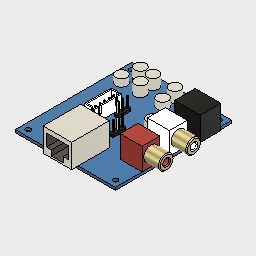
Rock64 ES9023 audio POT (Autodesk Fusion 360 design; units mm, degrees)
Autodesk Fusion 360 part; units mm, degrees
sketch "Sketch1" plane through (0, 0, 0) normal (0, 1, 0) x (1, 0, 0)
  line L0 (28.05, -32.6) -> (-28.05, -32.6)
  line L1 (-28.05, -32.6) -> (-28.05, 32.6)
  line L2 (-28.05, 32.6) -> (28.05, 32.6)
  line L3 (28.05, 32.6) -> (28.05, -32.6)
  line L4 (2.5, 0) -> (20, 0)
  line L5 (0, -20) -> (0, -2.5)
  circle A0 centre (-24.45, 29) radius 1.375
  circle A1 centre (24.55, 29) radius 1.375
  circle A2 centre (24.55, -29) radius 1.375
  circle A3 centre (-24.45, -29) radius 1.375
  dimension "d1" = 65.2
  dimension "d2" = 56.1
  dimension "d3" = 49
  dimension "d4" = 58
  dimension "d5" = 2.75
  dimension "d6" = 3.6
  dimension "d7" = 3.6
  measures "d1" distance of L0 L2
  measures "d2" distance of L1 L3
  measures "d3" distance of A0.centre A1.centre
  measures "d4" distance of A0.centre A3.centre
  measures "d5" diameter of A0
  measures "d6" distance of L0 A3.centre
  measures "d7" distance of L1 A3.centre
extrude "Extrude1" add sketch "Sketch1" along normal blind 1.5
sketch "Sketch2" plane through (0, 1.5, 0) normal (0, 1, 0) x (-1, 0, 0)
  circle A0 centre (24.45, 29) radius 1.375
  circle A1 centre (-24.55, 29) radius 1.375
  circle A2 centre (-24.55, -29) radius 1.375
  circle A3 centre (24.45, -29) radius 1.375
  line L0 (-28.05, -32.6) -> (28.05, -32.6)
  line L1 (28.05, -32.6) -> (28.05, 32.6)
  line L2 (28.05, 32.6) -> (-28.05, 32.6)
  line L3 (-28.05, 32.6) -> (-28.05, -32.6)
  line L4 (8.8, 15.2) -> (-7.2, 15.2)
  line L5 (-7.2, 15.2) -> (-7.2, 36.3)
  line L6 (-7.2, 36.3) -> (8.8, 36.3)
  line L7 (8.8, 36.3) -> (8.8, 15.2)
  dimension "d10" = 16
  dimension "d11" = 21.1
  dimension "d12" = 35.25
  dimension "d13" = 3.7
  measures "d10" distance of L5 L7
  measures "d11" distance of L4 L6
  measures "d12" distance of L1 L5
  measures "d13" distance of L2 L6
extrude "Extrude2" add sketch "Sketch2" along normal blind 13.25 contours L2 L5 L6 L7 | L2 L4 L5 L7
sketch "Sketch3" plane through (0, 0, 36.3) normal (0, 0, 1) x (1, 0, 0)
  line L0 (-8.8, 1.5) -> (7.2, 1.5)
  line L1 (7.2, 1.5) -> (7.2, 14.75)
  line L2 (7.2, 14.75) -> (-8.8, 14.75)
  line L3 (-8.8, 14.75) -> (-8.8, 1.5)
  line L4 (-6.8, 12.25) -> (5.2, 12.25)
  line L5 (5.2, 12.25) -> (5.2, 5.5)
  line L6 (-6.8, 5.5) -> (-6.8, 12.25)
  line L7 (2.5, 5.5) -> (2.5, 2.5)
  line L8 (2.5, 2.5) -> (-4.1, 2.5)
  line L9 (-4.1, 2.5) -> (-4.1, 5.5)
  line L10 (5.2, 5.5) -> (2.5, 5.5)
  line L11 (-4.1, 5.5) -> (-6.8, 5.5)
  dimension "d16" = 2.5
  dimension "d17" = 2
  dimension "d18" = 2
  dimension "d19" = 1
  dimension "d20" = 4
  dimension "d21" = 6.6
  measures "d16" distance of L2 L4
  measures "d17" distance of L3 L6
  measures "d18" distance of L1 L5
  measures "d19" distance of L0 L8
  measures "d20" distance of L0 L11
  measures "d21" distance of L7 L9
extrude "Extrude3" cut sketch "Sketch3" against normal blind 15 contours L4 L5 L6 L7 L8 L9 L10 L11
sketch "Sketch4" plane through (0, 1.5, 0) normal (0, 1, 0) x (-1, 0, 0)
  line L0 (-7.2, 15.2) -> (-7.2, 32.6)
  line L1 (-7.2, 32.6) -> (-28.05, 32.6)
  line L2 (-28.05, 32.6) -> (-28.05, -32.6)
  line L3 (-28.05, -32.6) -> (28.05, -32.6)
  line L4 (28.05, -32.6) -> (28.05, 32.6)
  line L5 (28.05, 32.6) -> (8.8, 32.6)
  line L6 (8.8, 32.6) -> (8.8, 15.2)
  line L7 (8.8, 15.2) -> (-7.2, 15.2)
  circle A0 centre (24.45, 29) radius 1.375
  circle A1 centre (-24.55, 29) radius 1.375
  circle A2 centre (-24.55, -29) radius 1.375
  circle A3 centre (24.45, -29) radius 1.375
  line L8 (-15.74, -7.7) -> (-28.04, -7.7)
  line L9 (-28.04, -7.7) -> (-28.04, 2.3)
  line L10 (-28.04, 2.3) -> (-15.74, 2.3)
  line L11 (-15.74, 2.3) -> (-15.74, -7.7)
  line L12 (-15.74, 7.6) -> (-28.04, 7.6)
  line L13 (-28.04, 7.6) -> (-28.04, 17.6)
  line L14 (-28.04, 17.6) -> (-15.74, 17.6)
  line L15 (-15.74, 17.6) -> (-15.74, 7.6)
  dimension "d24" = 12.3
  dimension "d25" = 10
  dimension "d26" = 5.3
  dimension "d27" = 15
  dimension "d30" = 0.01
  measures "d24" distance of L9 L11
  measures "d25" distance of L8 L10
  measures "d26" distance of L10 L12
  measures "d27" distance of L1 L14
  measures "d30" distance of L2 L9
extrude "Extrude4" add sketch "Sketch4" along normal blind 12.42 contours L8 L9 L10 L11 | L12 L13 L14 L15
sketch "Sketch5" plane through (28.04, 0, 0) normal (1, 0, 0) x (0, 0, -1)
  line L0 (-2.3, 1.5) -> (7.7, 1.5)
  line L1 (7.7, 1.5) -> (7.7, 13.92)
  line L2 (7.7, 13.92) -> (-2.3, 13.92)
  line L3 (-2.3, 13.92) -> (-2.3, 1.5)
  circle A0 centre (2.7, 8.02) radius 4.1
  circle A1 centre (-12.6, 8.02) radius 4.1
  circle A2 centre (-12.6, 8.02) radius 1.7
  circle A3 centre (2.7, 8.02) radius 1.7
  line L4 (-17.6, 1.5) -> (-17.6, 13.92)
  dimension "d31" = 8.2
  dimension "d32" = 3.4
  dimension "d33" = 5
  dimension "d34" = 5
  dimension "d35" = 5.9
  measures "d31" diameter of A1
  measures "d32" diameter of A2
  measures "d33" distance of A1.centre L4
  measures "d34" distance of L3 A0.centre
  measures "d35" distance of L2 A0.centre
extrude "Extrude5" add sketch "Sketch5" along normal blind 8.75 contours A0 | A1
fillet "Fillet1" radius 0.5 4 edges at (36.79, 6.5374, 16.4225) (36.79, 8.6347, 14.185) (36.79, 6.5374, 1.1225) (36.79, 8.6347, -1.115)
sketch "Sketch6" plane through (0, 1.5, 0) normal (0, 1, 0) x (-1, 0, 0)
  line L0 (-15.74, 17.6) -> (-15.74, 7.6)
  line L1 (-15.74, 7.6) -> (-28.04, 7.6)
  line L2 (-28.04, 7.6) -> (-28.04, 17.6)
  line L3 (-28.04, 17.6) -> (-15.74, 17.6)
  line L4 (-15.74, 2.3) -> (-15.74, -7.7)
  line L5 (-15.74, -7.7) -> (-28.04, -7.7)
  line L6 (-28.04, -7.7) -> (-28.04, 2.3)
  line L7 (-28.04, 2.3) -> (-15.74, 2.3)
  line L8 (-7.2, 15.2) -> (-7.2, 32.6)
  line L9 (-7.2, 32.6) -> (-28.05, 32.6)
  line L10 (-28.05, 32.6) -> (-28.05, -32.6)
  line L11 (-28.05, -32.6) -> (28.05, -32.6)
  line L12 (28.05, -32.6) -> (28.05, 32.6)
  line L13 (28.05, 32.6) -> (8.8, 32.6)
  line L14 (8.8, 32.6) -> (8.8, 15.2)
  line L15 (8.8, 15.2) -> (-7.2, 15.2)
  circle A0 centre (24.45, 29) radius 1.375
  circle A1 centre (-24.55, 29) radius 1.375
  circle A2 centre (-24.55, -29) radius 1.375
  circle A3 centre (24.45, -29) radius 1.375
  line L16 (-15.75, -24.5) -> (-30.05, -24.5)
  line L17 (-30.05, -24.5) -> (-30.05, -12.9)
  line L18 (-30.05, -12.9) -> (-15.75, -12.9)
  line L19 (-15.75, -12.9) -> (-15.75, -24.5)
  dimension "d39" = 11.6
  dimension "d40" = 14.3
  dimension "d41" = 2
  dimension "d42" = 8.1
  measures "d39" distance of L16 L18
  measures "d40" distance of L17 L19
  measures "d41" distance of L10 L17
  measures "d42" distance of L11 L16
extrude "Extrude6" add sketch "Sketch6" along normal blind 13.3 contours L10 L16 L18 L19 | L10 L16 L17 L18
sketch "Sketch7" plane through (0, 0, 0) normal (0, -1, 0) x (1, 0, 0)
  circle A0 centre (-24.45, 29) radius 1.375
  circle A1 centre (24.55, 29) radius 1.375
  circle A2 centre (24.55, -29) radius 1.375
  circle A3 centre (-24.45, -29) radius 1.375
  line L0 (-28.05, -32.6) -> (28.05, -32.6)
  line L1 (28.05, -32.6) -> (28.05, 32.6)
  line L2 (28.05, 32.6) -> (-28.05, 32.6)
  line L3 (-28.05, 32.6) -> (-28.05, -32.6)
  line L4 (-21.35, 20.3) -> (-16.45, 20.3)
  line L5 (-16.45, 20.3) -> (-16.45, -8.1)
  line L6 (-16.45, -8.1) -> (-21.35, -8.1)
  line L7 (-21.35, -8.1) -> (-21.35, 20.3)
  dimension "d45" = 4.9
  dimension "d46" = 28.4
  dimension "d47" = 6.7
  dimension "d48" = 12.3
  measures "d45" distance of L5 L7
  measures "d46" distance of L4 L6
  measures "d47" distance of L3 L7
  measures "d48" distance of L2 L4
extrude "Extrude7" add sketch "Sketch7" along normal blind 8.6 contours L4 L5 L6 L7
sketch "Sketch8" plane through (0, -8.6, 0) normal (0, -1, 0) x (1, 0, 0)
  line L0 (-21.35, -8.1) -> (-16.45, -8.1)
  line L1 (-16.45, -8.1) -> (-16.45, 20.3)
  line L2 (-16.45, 20.3) -> (-21.35, 20.3)
  line L3 (-21.35, 20.3) -> (-21.35, -8.1)
  line L4 (-20.49, 19.13) -> (-19.85, 19.13)
  line L5 (-19.85, 19.13) -> (-19.85, 18.49)
  line L6 (-19.85, 18.49) -> (-20.49, 18.49)
  line L7 (-20.49, 18.49) -> (-20.49, 19.13)
  dimension "d54" = 0.64
  dimension "d55" = 0.64
  dimension "d56" = 1.17
  dimension "d57" = 0.86
  measures "d54" distance of L4 L6
  measures "d55" distance of L5 L7
  measures "d56" distance of L2 L4
  measures "d57" distance of L3 L7
extrude "Extrude8" cut sketch "Sketch8" against normal blind 8 contours L4 L5 L6 L7
chamfer "Chamfer1" distance 0.55 angle 45 4 edges at (-19.85, -8.6, 18.81) (-20.17, -8.6, 19.13) (-20.49, -8.6, 18.81) (-20.17, -8.6, 18.49)
pattern_linear "R-Pattern1" count 2 spacing 2.54 along (1, 0, 0) count 11 spacing 2.54 along (0, 0, -1) of 9 faces at (-20.2767, -8.4167, 19.4967) (-20.8567, -8.4167, 18.9167) (-20.0633, -8.4167, 18.1233) (-19.4833, -8.4167, 18.9167) (-20.2767, -0.6, 18.9167) (-19.85, -5.5667, 18.9167) (-20.0633, -3.0833, 19.13) (-20.49, -5.5667, 18.7033) (-20.0633, -5.5667, 18.49)
sketch "Sketch9" plane through (0, 1.5, 0) normal (0, 1, 0) x (-1, 0, 0)
  line L0 (-15.75, -24.5) -> (-28.05, -24.5)
  line L1 (-28.05, -24.5) -> (-28.05, -32.6)
  line L2 (-28.05, -32.6) -> (28.05, -32.6)
  line L3 (28.05, -32.6) -> (28.05, 32.6)
  line L4 (28.05, 32.6) -> (8.8, 32.6)
  line L5 (8.8, 32.6) -> (8.8, 15.2)
  line L6 (8.8, 15.2) -> (-7.2, 15.2)
  line L7 (-7.2, 15.2) -> (-7.2, 32.6)
  line L8 (-7.2, 32.6) -> (-28.05, 32.6)
  line L9 (-28.05, 32.6) -> (-28.05, -12.9)
  line L10 (-28.05, -12.9) -> (-15.75, -12.9)
  line L11 (-15.75, -12.9) -> (-15.75, -24.5)
  line L12 (-15.74, 17.6) -> (-15.74, 7.6)
  line L13 (-15.74, 7.6) -> (-28.04, 7.6)
  line L14 (-28.04, 7.6) -> (-28.04, 17.6)
  line L15 (-28.04, 17.6) -> (-15.74, 17.6)
  line L16 (-15.74, 2.3) -> (-15.74, -7.7)
  line L17 (-15.74, -7.7) -> (-28.04, -7.7)
  line L18 (-28.04, -7.7) -> (-28.04, 2.3)
  line L19 (-28.04, 2.3) -> (-15.74, 2.3)
  circle A0 centre (24.45, 29) radius 1.375
  circle A1 centre (-24.55, 29) radius 1.375
  circle A2 centre (-24.55, -29) radius 1.375
  circle A3 centre (24.45, -29) radius 1.375
  line L20 (18.5, -7.46) -> (18.5, -5.72)
  line L21 (18.5, -5.72) -> (16.76, -5.72)
  line L22 (16.76, -5.72) -> (16.76, -7.46)
  line L23 (16.76, -7.46) -> (18.5, -7.46)
  line L24 (21.04, -7.46) -> (21.04, -5.72)
  line L25 (21.04, -5.72) -> (19.3, -5.72)
  line L26 (19.3, -5.72) -> (19.3, -7.46)
  line L27 (19.3, -7.46) -> (21.04, -7.46)
  line L28 (18.5, -4.92) -> (18.5, -3.18)
  line L29 (18.5, -3.18) -> (16.76, -3.18)
  line L30 (16.76, -3.18) -> (16.76, -4.92)
  line L31 (16.76, -4.92) -> (18.5, -4.92)
  line L32 (21.04, -4.92) -> (21.04, -3.18)
  line L33 (21.04, -3.18) -> (19.3, -3.18)
  line L34 (19.3, -3.18) -> (19.3, -4.92)
  line L35 (19.3, -4.92) -> (21.04, -4.92)
  line L36 (18.5, -2.38) -> (18.5, -0.64)
  line L37 (18.5, -0.64) -> (16.76, -0.64)
  line L38 (16.76, -0.64) -> (16.76, -2.38)
  line L39 (16.76, -2.38) -> (18.5, -2.38)
  line L40 (21.04, -2.38) -> (21.04, -0.64)
  line L41 (21.04, -0.64) -> (19.3, -0.64)
  line L42 (19.3, -0.64) -> (19.3, -2.38)
  line L43 (19.3, -2.38) -> (21.04, -2.38)
  line L44 (18.5, 0.16) -> (18.5, 1.9)
  line L45 (18.5, 1.9) -> (16.76, 1.9)
  line L46 (16.76, 1.9) -> (16.76, 0.16)
  line L47 (16.76, 0.16) -> (18.5, 0.16)
  line L48 (21.04, 0.16) -> (21.04, 1.9)
  line L49 (21.04, 1.9) -> (19.3, 1.9)
  line L50 (19.3, 1.9) -> (19.3, 0.16)
  line L51 (19.3, 0.16) -> (21.04, 0.16)
  line L52 (18.5, 2.7) -> (18.5, 4.44)
  line L53 (18.5, 4.44) -> (16.76, 4.44)
  line L54 (16.76, 4.44) -> (16.76, 2.7)
  line L55 (16.76, 2.7) -> (18.5, 2.7)
  line L56 (21.04, 2.7) -> (21.04, 4.44)
  line L57 (21.04, 4.44) -> (19.3, 4.44)
  line L58 (19.3, 4.44) -> (19.3, 2.7)
  line L59 (19.3, 2.7) -> (21.04, 2.7)
  line L60 (18.5, 5.24) -> (18.5, 6.98)
  line L61 (18.5, 6.98) -> (16.76, 6.98)
  line L62 (16.76, 6.98) -> (16.76, 5.24)
  line L63 (16.76, 5.24) -> (18.5, 5.24)
  line L64 (21.04, 5.24) -> (21.04, 6.98)
  line L65 (21.04, 6.98) -> (19.3, 6.98)
  line L66 (19.3, 6.98) -> (19.3, 5.24)
  line L67 (19.3, 5.24) -> (21.04, 5.24)
  line L68 (18.5, 7.78) -> (18.5, 9.52)
  line L69 (18.5, 9.52) -> (16.76, 9.52)
  line L70 (16.76, 9.52) -> (16.76, 7.78)
  line L71 (16.76, 7.78) -> (18.5, 7.78)
  line L72 (21.04, 7.78) -> (21.04, 9.52)
  line L73 (21.04, 9.52) -> (19.3, 9.52)
  line L74 (19.3, 9.52) -> (19.3, 7.78)
  line L75 (19.3, 7.78) -> (21.04, 7.78)
  line L76 (18.5, 10.32) -> (18.5, 12.06)
  line L77 (18.5, 12.06) -> (16.76, 12.06)
  line L78 (16.76, 12.06) -> (16.76, 10.32)
  line L79 (16.76, 10.32) -> (18.5, 10.32)
  line L80 (21.04, 10.32) -> (21.04, 12.06)
  line L81 (21.04, 12.06) -> (19.3, 12.06)
  line L82 (19.3, 12.06) -> (19.3, 10.32)
  line L83 (19.3, 10.32) -> (21.04, 10.32)
  line L84 (18.5, 12.86) -> (18.5, 14.6)
  line L85 (18.5, 14.6) -> (16.76, 14.6)
  line L86 (16.76, 14.6) -> (16.76, 12.86)
  line L87 (16.76, 12.86) -> (18.5, 12.86)
  line L88 (21.04, 12.86) -> (21.04, 14.6)
  line L89 (21.04, 14.6) -> (19.3, 14.6)
  line L90 (19.3, 14.6) -> (19.3, 12.86)
  line L91 (19.3, 12.86) -> (21.04, 12.86)
  line L92 (18.5, 15.4) -> (18.5, 17.14)
  line L93 (18.5, 17.14) -> (16.76, 17.14)
  line L94 (16.76, 17.14) -> (16.76, 15.4)
  line L95 (16.76, 15.4) -> (18.5, 15.4)
  line L96 (21.04, 15.4) -> (21.04, 17.14)
  line L97 (21.04, 17.14) -> (19.3, 17.14)
  line L98 (19.3, 17.14) -> (19.3, 15.4)
  line L99 (19.3, 15.4) -> (21.04, 15.4)
  line L100 (18.5, 17.94) -> (18.5, 19.68)
  line L101 (18.5, 19.68) -> (16.76, 19.68)
  line L102 (16.76, 19.68) -> (16.76, 17.94)
  line L103 (16.76, 17.94) -> (18.5, 17.94)
  line L104 (21.35, -8.1) -> (16.45, -8.1)
  line L105 (16.45, -8.1) -> (16.45, 20.3)
  line L106 (16.45, 20.3) -> (21.35, 20.3)
  line L107 (21.35, 20.3) -> (21.35, -8.1)
  line L108 (19.3, 19.68) -> (19.3, 17.94)
  line L109 (19.3, 17.94) -> (21.04, 17.94)
  line L110 (21.04, 17.94) -> (21.04, 19.68)
  line L111 (21.04, 19.68) -> (19.3, 19.68)
  circle A4 centre (20.17, -6.59) radius 0.635
  point P0 (20.17, -6.59)
  dimension "d77" = 1.27
  measures "d77" diameter of A4
extrude "Extrude10" add sketch "Sketch9" along normal blind 0.7 contours A4
fillet "Fillet4" radius 0.6 1 edges at (-19.578, 2.2, -6.8196)
pattern_linear "R-Pattern3" count 2 spacing 2.54 along (1, 0, 0) count 11 spacing 2.54 along (0, 0, 1) of 3 faces at (-20.1604, 2.2, -6.6) (-20.7491, 1.823, -6.4669) (-20.8042, 1.5667, -6.6217)
sketch "Sketch10" plane through (0, 1.5, 0) normal (0, 1, 0) x (-1, 0, 0)
  line L0 (8.5, 7.6) -> (14.25, 7.6)
  line L1 (14.25, 7.6) -> (14.25, -7.4)
  line L2 (14.25, -7.4) -> (8.5, -7.4)
  line L3 (8.5, -7.4) -> (8.5, 7.6)
  line L4 (28.05, -32.6) -> (28.05, 32.6)
  line L5 (28.05, 32.6) -> (8.8, 32.6)
  line L6 (13.5, -6.65) -> (9.25, -6.65)
  line L7 (9.25, -6.65) -> (9.25, 6.85)
  line L8 (9.25, 6.85) -> (13.5, 6.85)
  line L9 (13.5, 6.85) -> (13.5, -6.65)
  dimension "d83" = 0.75
  dimension "d104" = 15
  dimension "d105" = 5.75
  dimension "d106" = 13.8
  dimension "d107" = 25
  measures "d104" distance of L0 L2
  measures "d105" distance of L1 L3
  measures "d106" distance of L1 L4
  measures "d107" distance of L0 L5
extrude "Extrude11" add sketch "Sketch10" along normal blind 7.1
sketch "Sketch11" plane through (0, 1.5, 0) normal (0, 1, 0) x (-1, 0, 0)
  line L0 (9.25, 6.85) -> (9.25, -6.65)
  line L1 (9.25, -6.65) -> (13.5, -6.65)
  line L2 (13.5, -6.65) -> (13.5, 6.85)
  line L3 (13.5, 6.85) -> (9.25, 6.85)
  line L4 (11, -5.55) -> (10.35, -5.55)
  line L5 (10.35, -5.55) -> (10.35, -4.9)
  line L6 (10.35, -4.9) -> (11, -4.9)
  line L7 (11, -4.9) -> (11, -5.55)
  dimension "d86" = 1.1
  dimension "d87" = 0.65
  dimension "d88" = 0.65
  dimension "d89" = 1.1
  measures "d86" distance of L0 L5
  measures "d87" distance of L4.end L5.end
  measures "d88" distance of L4.start L4.end
  measures "d89" distance of L1 L4
extrude "Extrude12" add sketch "Sketch11" along normal blind 6.5 contours L4 L5 L6 L7
sketch "Sketch12" plane through (0, 8.6, 0) normal (0, 1, 0) x (-1, 0, 0)
  line L0 (9.25, 6.85) -> (13.5, 6.85)
  line L1 (13.5, 6.85) -> (13.5, -6.65)
  line L2 (13.5, -6.65) -> (9.25, -6.65)
  line L3 (9.25, -6.65) -> (9.25, 6.85)
  line L4 (8.5, -7.4) -> (14.25, -7.4)
  line L5 (14.25, -7.4) -> (14.25, 7.6)
  line L6 (14.25, 7.6) -> (8.5, 7.6)
  line L7 (8.5, 7.6) -> (8.5, -7.4)
  line L8 (9.25, -6.65) -> (10.35, -6.65)
  line L9 (10.35, -6.65) -> (10.35, -7.4)
  line L10 (10.35, -7.4) -> (9.25, -7.4)
  line L11 (9.25, -7.4) -> (9.25, -6.65)
  line L12 (9.25, -5.2) -> (8.5, -5.2)
  line L13 (8.5, -5.2) -> (8.5, -3.9)
  line L14 (8.5, -3.9) -> (9.25, -3.9)
  line L15 (9.25, -3.9) -> (9.25, -5.2)
  line L16 (8.5, 5.4) -> (9.25, 5.4)
  line L17 (9.25, 5.4) -> (9.25, 4.1)
  line L18 (9.25, 4.1) -> (8.5, 4.1)
  line L19 (8.5, 4.1) -> (8.5, 5.4)
  line L20 (9.25, 6.85) -> (10.35, 6.85)
  line L21 (10.35, 6.85) -> (10.35, 7.6)
  line L22 (10.35, 7.6) -> (9.25, 7.6)
  line L23 (9.25, 7.6) -> (9.25, 6.85)
  dimension "d92" = 1.1
  dimension "d93" = 1.1
  dimension "d94" = 2.2
  dimension "d95" = 1.3
  dimension "d96" = 2.2
  dimension "d97" = 1.3
  measures "d92" distance of L2.end L8.end
  measures "d93" distance of L21 L23
  measures "d94" distance of L6 L16
  measures "d95" distance of L16 L18
  measures "d96" distance of L4 L12
  measures "d97" distance of L12 L14
extrude "Extrude13" cut sketch "Sketch12" against normal blind 4 contours L0 L6 L20 L21 L22 L23 | L3 L7 L16 L17 L18 L19 | L3 L7 L12 L13 L14 L15 | L2 L4 L8 L9 L10 L11
pattern_linear "R-Pattern4" count 5 spacing 2.54 along (0, 0, 1) of "Extrude12"
sketch "Sketch14" plane through (0, 1.5, 0) normal (0, 1, 0) x (-1, 0, 0)
  circle A0 centre (24.45, -29) radius 1.375
  circle A1 centre (-24.55, -29) radius 1.375
  circle A2 centre (-24.55, 29) radius 1.375
  circle A3 centre (24.45, 29) radius 1.375
  line L0 (-15.74, 2.3) -> (-15.74, -7.7)
  line L1 (-15.74, -7.7) -> (-28.04, -7.7)
  line L2 (-28.04, -7.7) -> (-28.04, 2.3)
  line L3 (-28.04, 2.3) -> (-15.74, 2.3)
  line L4 (-15.74, 17.6) -> (-15.74, 7.6)
  line L5 (-15.74, 7.6) -> (-28.04, 7.6)
  line L6 (-28.04, 7.6) -> (-28.04, 17.6)
  line L7 (-28.04, 17.6) -> (-15.74, 17.6)
  line L8 (-15.75, -24.5) -> (-28.05, -24.5)
  line L9 (-28.05, -24.5) -> (-28.05, -32.6)
  line L10 (-28.05, -32.6) -> (28.05, -32.6)
  line L11 (28.05, -32.6) -> (28.05, 32.6)
  line L12 (28.05, 32.6) -> (8.8, 32.6)
  line L13 (8.8, 32.6) -> (8.8, 15.2)
  line L14 (8.8, 15.2) -> (-7.2, 15.2)
  line L15 (-7.2, 15.2) -> (-7.2, 32.6)
  line L16 (-7.2, 32.6) -> (-28.05, 32.6)
  line L17 (-28.05, 32.6) -> (-28.05, -12.9)
  line L18 (-28.05, -12.9) -> (-15.75, -12.9)
  line L19 (-15.75, -12.9) -> (-15.75, -24.5)
  circle A4 centre (20.17, -6.59) radius 0.635
  circle A5 centre (17.63, -6.59) radius 0.635
  circle A6 centre (20.17, -4.05) radius 0.635
  circle A7 centre (17.63, -4.05) radius 0.635
  circle A8 centre (20.17, -1.51) radius 0.635
  circle A9 centre (17.63, -1.51) radius 0.635
  circle A10 centre (20.17, 1.03) radius 0.635
  circle A11 centre (17.63, 1.03) radius 0.635
  circle A12 centre (20.17, 3.57) radius 0.635
  circle A13 centre (17.63, 3.57) radius 0.635
  circle A14 centre (20.17, 6.11) radius 0.635
  circle A15 centre (17.63, 6.11) radius 0.635
  circle A16 centre (20.17, 8.65) radius 0.635
  circle A17 centre (17.63, 8.65) radius 0.635
  circle A18 centre (20.17, 11.19) radius 0.635
  circle A19 centre (17.63, 11.19) radius 0.635
  circle A20 centre (20.17, 13.73) radius 0.635
  circle A21 centre (17.63, 13.73) radius 0.635
  circle A22 centre (20.17, 16.27) radius 0.635
  circle A23 centre (17.63, 16.27) radius 0.635
  circle A24 centre (20.17, 18.81) radius 0.635
  circle A25 centre (17.63, 18.81) radius 0.635
  line L20 (8.5, -7.4) -> (8.5, 7.6)
  line L21 (8.5, 7.6) -> (14.25, 7.6)
  line L22 (14.25, 7.6) -> (14.25, -7.4)
  line L23 (14.25, -7.4) -> (8.5, -7.4)
  line L24 (7.05, -9.1) -> (4.65, -9.1)
  line L25 (4.65, -9.1) -> (4.65, -1.32)
  line L26 (4.65, -1.32) -> (7.05, -1.32)
  line L27 (7.05, -1.32) -> (7.05, -9.1)
  line L28 (-0.95, 1.42) -> (-3.35, 1.42)
  line L29 (-3.35, 1.42) -> (-3.35, 9.2)
  line L30 (-3.35, 9.2) -> (-0.95, 9.2)
  line L31 (-0.95, 9.2) -> (-0.95, 1.42)
  dimension "d108" = 2.4
  dimension "d109" = 7.78
  dimension "d110" = 6
  dimension "d111" = 24.7
  dimension "d112" = 21
  dimension "d113" = 23.5
  measures "d108" distance of L25 L27
  measures "d109" distance of L24 L26
  measures "d110" distance of L14 L30
  measures "d111" distance of L17 L29
  measures "d112" distance of L11 L27
  measures "d113" distance of L10 L24
extrude "Extrude14" add sketch "Sketch14" along normal blind 1.3 contours L24 L25 L26 L27 | L28 L29 L30 L31
chamfer "Chamfer2" distance 0.65 angle 45 8 edges at (-7.05, 2.15, -9.1) (-4.65, 2.15, -9.1) (0.95, 2.15, 1.42) (3.35, 2.15, 1.42) (-7.05, 2.15, -1.32) (-4.65, 2.15, -1.32) (3.35, 2.15, 9.2) (0.95, 2.15, 9.2)
sketch "Sketch15" plane through (0, 2.8, 0) normal (0, 1, 0) x (-1, 0, 0)
  line L0 (5.3, -1.32) -> (4.65, -1.97)
  line L1 (4.65, -1.97) -> (4.65, -8.45)
  line L2 (4.65, -8.45) -> (5.3, -9.1)
  line L3 (5.3, -9.1) -> (6.4, -9.1)
  line L4 (6.4, -9.1) -> (7.05, -8.45)
  line L5 (7.05, -8.45) -> (7.05, -1.97)
  line L6 (7.05, -1.97) -> (6.4, -1.32)
  line L7 (6.4, -1.32) -> (5.3, -1.32)
  line L8 (6.17, -8.22) -> (5.52, -8.22)
  line L9 (5.52, -8.22) -> (5.52, -7.57)
  line L10 (5.52, -7.57) -> (6.17, -7.57)
  line L11 (6.17, -7.57) -> (6.17, -8.22)
  line L12 (-1.83, 2.3) -> (-2.48, 2.3)
  line L13 (-2.48, 2.3) -> (-2.48, 2.95)
  line L14 (-2.48, 2.95) -> (-1.83, 2.95)
  line L15 (-1.83, 2.95) -> (-1.83, 2.3)
  line L16 (-0.95, 2.07) -> (-0.95, 8.55)
  line L17 (-2.7, 1.42) -> (-1.6, 1.42)
  dimension "d117" = 0.65
  dimension "d118" = 0.88
  dimension "d119" = 0.88
  dimension "d120" = 0.88
  dimension "d121" = 0.88
  measures "d117" distance of L9 L11
  measures "d118" distance of L5 L11
  measures "d119" distance of L3 L8
  measures "d120" distance of L15 L16
  measures "d121" distance of L12 L17
extrude "Extrude15" add sketch "Sketch15" along normal blind 6 contours L8 L9 L10 L11 | L12 L13 L14 L15
pattern_linear "R-Pattern5" count 3 spacing 2.54 along (0, 0, 1) of "Extrude15"
sketch "Sketch16" plane through (0, 1.5, 0) normal (0, 1, 0) x (-1, 0, 0)
  line L0 (-0.95, 8.55) -> (-0.95, 2.07)
  line L1 (-0.95, 2.07) -> (-1.6, 1.42)
  line L2 (-1.6, 1.42) -> (-2.7, 1.42)
  line L3 (-2.7, 1.42) -> (-3.35, 2.07)
  line L4 (-3.35, 2.07) -> (-3.35, 8.55)
  line L5 (-3.35, 8.55) -> (-2.7, 9.2)
  line L6 (-2.7, 9.2) -> (-1.6, 9.2)
  line L7 (-1.6, 9.2) -> (-0.95, 8.55)
  line L8 (7.05, -1.97) -> (7.05, -8.45)
  line L9 (7.05, -8.45) -> (6.4, -9.1)
  line L10 (6.4, -9.1) -> (5.3, -9.1)
  line L11 (5.3, -9.1) -> (4.65, -8.45)
  line L12 (4.65, -8.45) -> (4.65, -1.97)
  line L13 (4.65, -1.97) -> (5.3, -1.32)
  line L14 (5.3, -1.32) -> (6.4, -1.32)
  line L15 (6.4, -1.32) -> (7.05, -1.97)
  circle A0 centre (24.45, -29) radius 1.375
  circle A1 centre (-24.55, -29) radius 1.375
  circle A2 centre (-24.55, 29) radius 1.375
  circle A3 centre (24.45, 29) radius 1.375
  line L16 (-15.74, 2.3) -> (-15.74, -7.7)
  line L17 (-15.74, -7.7) -> (-28.04, -7.7)
  line L18 (-28.04, -7.7) -> (-28.04, 2.3)
  line L19 (-28.04, 2.3) -> (-15.74, 2.3)
  line L20 (-15.74, 17.6) -> (-15.74, 7.6)
  line L21 (-15.74, 7.6) -> (-28.04, 7.6)
  line L22 (-28.04, 7.6) -> (-28.04, 17.6)
  line L23 (-28.04, 17.6) -> (-15.74, 17.6)
  line L24 (-15.75, -24.5) -> (-28.05, -24.5)
  line L25 (-28.05, -24.5) -> (-28.05, -32.6)
  line L26 (-28.05, -32.6) -> (28.05, -32.6)
  line L27 (28.05, -32.6) -> (28.05, 32.6)
  line L28 (28.05, 32.6) -> (8.8, 32.6)
  line L29 (8.8, 32.6) -> (8.8, 15.2)
  line L30 (8.8, 15.2) -> (-7.2, 15.2)
  line L31 (-7.2, 15.2) -> (-7.2, 32.6)
  line L32 (-7.2, 32.6) -> (-28.05, 32.6)
  line L33 (-28.05, 32.6) -> (-28.05, -12.9)
  line L34 (-28.05, -12.9) -> (-15.75, -12.9)
  line L35 (-15.75, -12.9) -> (-15.75, -24.5)
  circle A4 centre (20.17, -6.59) radius 0.635
  circle A5 centre (17.63, -6.59) radius 0.635
  circle A6 centre (20.17, -4.05) radius 0.635
  circle A7 centre (17.63, -4.05) radius 0.635
  circle A8 centre (20.17, -1.51) radius 0.635
  circle A9 centre (17.63, -1.51) radius 0.635
  circle A10 centre (20.17, 1.03) radius 0.635
  circle A11 centre (17.63, 1.03) radius 0.635
  circle A12 centre (20.17, 3.57) radius 0.635
  circle A13 centre (17.63, 3.57) radius 0.635
  circle A14 centre (20.17, 6.11) radius 0.635
  circle A15 centre (17.63, 6.11) radius 0.635
  circle A16 centre (20.17, 8.65) radius 0.635
  circle A17 centre (17.63, 8.65) radius 0.635
  circle A18 centre (20.17, 11.19) radius 0.635
  circle A19 centre (17.63, 11.19) radius 0.635
  circle A20 centre (20.17, 13.73) radius 0.635
  circle A21 centre (17.63, 13.73) radius 0.635
  circle A22 centre (20.17, 16.27) radius 0.635
  circle A23 centre (17.63, 16.27) radius 0.635
  circle A24 centre (20.17, 18.81) radius 0.635
  circle A25 centre (17.63, 18.81) radius 0.635
  line L36 (8.5, -7.4) -> (8.5, 7.6)
  line L37 (8.5, 7.6) -> (14.25, 7.6)
  line L38 (14.25, 7.6) -> (14.25, -7.4)
  line L39 (14.25, -7.4) -> (8.5, -7.4)
  circle A26 centre (-1.8, -27.15) radius 3.15
  circle A27 centre (10.7, -27.15) radius 3.15
  circle A28 centre (17.7, -27.15) radius 3.15
  circle A29 centre (10.7, -20.15) radius 3.15
  circle A30 centre (-10.74, -5.45) radius 3.15
  dimension "d128" = 6.3
  dimension "d129" = 10.35
  dimension "d130" = 7
  dimension "d131" = 7
  dimension "d132" = 12.5
  dimension "d133" = 5.45
  dimension "d136" = 27.15
  dimension "d138" = 5
  measures "d128" diameter of A27
  measures "d129" distance of L27 A28.centre
  measures "d130" distance of A27.centre A28.centre
  measures "d131" distance of A27.centre A29.centre
  measures "d132" distance of A26.centre A27.centre
  measures "d133" distance of L26 A28.centre
  measures "d136" distance of L26 A30.centre
  measures "d138" distance of L16 A30.centre
extrude "Extrude16" add sketch "Sketch16" along normal blind 5.8 contours A26 | A27 | A28 | A29 | A30
sketch "Sketch18" plane through (0, 1.5, 0) normal (0, 1, 0) x (-1, 0, 0)
  circle A0 centre (-10.74, -5.45) radius 3.15
  circle A1 centre (17.7, -27.15) radius 3.15
  circle A2 centre (-1.8, -27.15) radius 3.15
  circle A3 centre (10.7, -27.15) radius 3.15
  circle A4 centre (10.7, -20.15) radius 3.15
  line L0 (-0.95, 8.55) -> (-0.95, 2.07)
  line L1 (-0.95, 2.07) -> (-1.6, 1.42)
  line L2 (-1.6, 1.42) -> (-2.7, 1.42)
  line L3 (-2.7, 1.42) -> (-3.35, 2.07)
  line L4 (-3.35, 2.07) -> (-3.35, 8.55)
  line L5 (-3.35, 8.55) -> (-2.7, 9.2)
  line L6 (-2.7, 9.2) -> (-1.6, 9.2)
  line L7 (-1.6, 9.2) -> (-0.95, 8.55)
  line L8 (7.05, -1.97) -> (7.05, -8.45)
  line L9 (7.05, -8.45) -> (6.4, -9.1)
  line L10 (6.4, -9.1) -> (5.3, -9.1)
  line L11 (5.3, -9.1) -> (4.65, -8.45)
  line L12 (4.65, -8.45) -> (4.65, -1.97)
  line L13 (4.65, -1.97) -> (5.3, -1.32)
  line L14 (5.3, -1.32) -> (6.4, -1.32)
  line L15 (6.4, -1.32) -> (7.05, -1.97)
  circle A5 centre (24.45, -29) radius 1.375
  circle A6 centre (-24.55, -29) radius 1.375
  circle A7 centre (-24.55, 29) radius 1.375
  circle A8 centre (24.45, 29) radius 1.375
  line L16 (-15.74, 2.3) -> (-15.74, -7.7)
  line L17 (-15.74, -7.7) -> (-28.04, -7.7)
  line L18 (-28.04, -7.7) -> (-28.04, 2.3)
  line L19 (-28.04, 2.3) -> (-15.74, 2.3)
  line L20 (-15.74, 17.6) -> (-15.74, 7.6)
  line L21 (-15.74, 7.6) -> (-28.04, 7.6)
  line L22 (-28.04, 7.6) -> (-28.04, 17.6)
  line L23 (-28.04, 17.6) -> (-15.74, 17.6)
  line L24 (-15.75, -24.5) -> (-28.05, -24.5)
  line L25 (-28.05, -24.5) -> (-28.05, -32.6)
  line L26 (-28.05, -32.6) -> (28.05, -32.6)
  line L27 (28.05, -32.6) -> (28.05, 32.6)
  line L28 (28.05, 32.6) -> (8.8, 32.6)
  line L29 (8.8, 32.6) -> (8.8, 15.2)
  line L30 (8.8, 15.2) -> (-7.2, 15.2)
  line L31 (-7.2, 15.2) -> (-7.2, 32.6)
  line L32 (-7.2, 32.6) -> (-28.05, 32.6)
  line L33 (-28.05, 32.6) -> (-28.05, -12.9)
  line L34 (-28.05, -12.9) -> (-15.75, -12.9)
  line L35 (-15.75, -12.9) -> (-15.75, -24.5)
  circle A9 centre (20.17, -6.59) radius 0.635
  circle A10 centre (17.63, -6.59) radius 0.635
  circle A11 centre (20.17, -4.05) radius 0.635
  circle A12 centre (17.63, -4.05) radius 0.635
  circle A13 centre (20.17, -1.51) radius 0.635
  circle A14 centre (17.63, -1.51) radius 0.635
  circle A15 centre (20.17, 1.03) radius 0.635
  circle A16 centre (17.63, 1.03) radius 0.635
  circle A17 centre (20.17, 3.57) radius 0.635
  circle A18 centre (17.63, 3.57) radius 0.635
  circle A19 centre (20.17, 6.11) radius 0.635
  circle A20 centre (17.63, 6.11) radius 0.635
  circle A21 centre (20.17, 8.65) radius 0.635
  circle A22 centre (17.63, 8.65) radius 0.635
  circle A23 centre (20.17, 11.19) radius 0.635
  circle A24 centre (17.63, 11.19) radius 0.635
  circle A25 centre (20.17, 13.73) radius 0.635
  circle A26 centre (17.63, 13.73) radius 0.635
  circle A27 centre (20.17, 16.27) radius 0.635
  circle A28 centre (17.63, 16.27) radius 0.635
  circle A29 centre (20.17, 18.81) radius 0.635
  circle A30 centre (17.63, 18.81) radius 0.635
  line L36 (8.5, -7.4) -> (8.5, 7.6)
  line L37 (8.5, 7.6) -> (14.25, 7.6)
  line L38 (14.25, 7.6) -> (14.25, -7.4)
  line L39 (14.25, -7.4) -> (8.5, -7.4)
  circle A31 centre (-1.8, -20.15) radius 3.15
  circle A32 centre (21.15, -19.95) radius 3.15
  dimension "d140" = 6.9
  dimension "d141" = 12.65
  measures "d140" distance of L27 A32.centre
  measures "d141" distance of L26 A32.centre
extrude "Extrude17" add sketch "Sketch18" along normal blind 4 contours A31 | A32
equation "d6 = 2.2 mm + 1.4 mm"
equation "d7 = 2.2 mm + 1.4 mm"
equation "d28 = 13.92 mm - 1.5 mm"
equation "d35 = 10 mm - ( ( 8.2 / 2 ) * 1 mm )"
equation "d56 = 0.96 mm + 0.21 mm"
equation "d118 = ( 2.4 / 2 ) * 1 mm - 0.32 mm"
equation "d129 = 7.2 mm + 3.15 mm"
equation "d132 = 6.2 mm + 6.3 mm"
equation "d133 = 2.3 mm + 3.15 mm"
equation "d136 = 24 mm + 3.15 mm"
equation "d140 = 3.75 mm + 3.15 mm"
equation "d141 = 9.5 mm + 3.15 mm"
